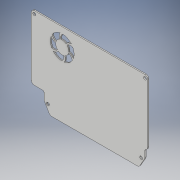
# Autodesk Inventor part: Back Plate
Saved by Autodesk Inventor 2019.4 (Build 234330000, 330)
## iProperties
Created: 2020-08-29
Part Number: Back Plate
Material: Generic
Document SubType Name: Modeling
Designer: craig
Density: 1 g/cm^3
Appearance: Default
Author: craig
Autodesk Inventor part; units mm, degrees
ref_plane "YZ Plane" through (0, 0, 0) normal (1, 0, 0) x (0, 1, 0)
ref_plane "XZ Plane" through (0, 0, 0) normal (0, 1, 0) x (-1, 0, 0)
ref_plane "XY Plane" through (0, 0, 0) normal (0, 0, 1) x (1, 0, 0)
sketch "Sketch4" plane through (0, 0, 0) normal (0, 0, 1) x (1, 0, 0)
  line L0 (92.7325, 70.7032) -> (-95.1675, 70.7032) projected
  arc A0 (-95.1675, 70.7032) -> (-99.1675, 66.7032) centre (-95.1675, 66.7032) ccw projected
  line L1 (-99.1675, 66.7032) -> (-99.1675, -37.2051) projected
  arc A1 (-91.7887, 67.4724) -> (-95.6675, 64.7032) centre (-94.1675, 66.7032) ccw projected
  line L2 (-99.1675, -37.2051) -> (-79.7175, -37.2051) projected
  arc A2 (-77.7175, -39.2051) -> (-79.7175, -37.2051) centre (-79.7175, -39.2051) ccw projected
  line L3 (-77.7175, -39.2051) -> (-77.7175, -50.6763) projected
  line L4 (-77.7175, -50.6763) -> (-67.7175, -67.9968) projected
  line L5 (-67.7175, -67.9968) -> (82.2825, -67.9968) projected
  circle A3 centre (-71.0649, -52.9681) radius 2.5 projected
  line L6 (82.2825, -67.9968) -> (92.2825, -50.6763) projected
  circle A4 centre (86.0549, -52.9681) radius 2.5 projected
  line L7 (92.2825, -50.6763) -> (92.2825, -39.2051) projected
  arc A5 (94.2825, -37.2051) -> (92.2825, -39.2051) centre (94.2825, -39.2051) ccw projected
  line L8 (94.2825, -37.2051) -> (96.7325, -37.2051) projected
  line L9 (96.7325, -37.2051) -> (96.7325, 66.7032) projected
  arc A6 (96.7325, 66.7032) -> (92.7325, 70.7032) centre (92.7325, 66.7032) ccw projected
  arc A7 (93.3598, 64.019) -> (90.8929, 68.2807) centre (92.5018, 66.3672) ccw projected
  arc A8 (90.8929, 68.2807) -> (93.3598, 64.019) centre (92.5018, 66.3672) ccw
  arc A9 (-95.6675, 64.7032) -> (-91.7887, 67.4724) centre (-94.1675, 66.7032) ccw
  point P0 (0, 0)
  constraints: 4 point on circle, 2 centre point, 2 concentric
extrude "Extrusion4" add sketch "Sketch4" along normal blind 2
fillet "Fillet1" radius 5 6 edges at (-99.1675, -37.2051, 1) (-77.7175, -50.6763, 1) (-67.7175, -67.9968, 1) (82.2825, -67.9968, 1) (92.2825, -50.6763, 1) (96.7325, -37.2051, 1)
sketch "Sketch5" plane through (0, 0, 2) normal (0, 0, 1) x (1, 0, 0)
  circle A0 centre (-46.9967, 41.5331) radius 20
  circle A1 centre (-46.9967, 41.5331) radius 11
  point P0 (0, 0)
  dimension "d12" = 40
  dimension "d13" = 22
  constraints: 2 centre point, 1 coincident
  measures "d12" diameter of A0
  measures "d13" diameter of A1
extrude "Extrusion5" cut sketch "Sketch5" against normal blind 10
sketch "Sketch6" plane through (0, 0, 2) normal (0, 0, 1) x (1, 0, 0)
  arc A0 (-46.4486, 64.74) -> (-47.34, 46.911) centre (-41.9812, 55.5798) ccw
  arc A1 (-38.695, 63.3) -> (-44.2546, 45.6452) centre (-40.3973, 54.1333) ccw
  line L0 (-47.34, 46.911) -> (-44.2546, 45.6452)
  line L1 (-46.4486, 64.74) -> (-38.695, 63.3)
  point P0 (0, 0)
  constraints: 4 end point, 4 point on circle, 2 centre point, 1 tangent
extrude "Extrusion6" add sketch "Sketch6" against normal up to surface (2 mm away)
pattern_circular "Circular Pattern1" count 6 over 360 about axis through (-46.9967, 41.5331, 2) along (0, 0, -1) of "Extrusion6"
sketch "Sketch7" plane through (0, 0, 2) normal (0, 0, 1) x (1, 0, 0)
  line L0 (-95.1675, 71.7032) -> (92.7325, 71.7032) projected
  line L1 (92.7325, 70.7032) -> (-95.1675, 70.7032) projected
  arc A0 (-95.1675, 70.7032) -> (-99.1675, 66.7032) centre (-95.1675, 66.7032) ccw projected
  arc A1 (-95.1675, 71.7032) -> (-99.1675, 66.7032) centre (-94.4287, 67.0121) ccw projected
  arc A2 (96.7325, 66.7032) -> (92.7325, 70.7032) centre (92.7325, 66.7032) ccw projected
  arc A3 (96.7325, 66.7032) -> (92.7325, 71.7032) centre (91.9937, 67.0121) ccw projected
  point P0 (0, 0)
extrude "Extrusion7" add sketch "Sketch7" against normal up to surface (2 mm away)
body "Solid2"
